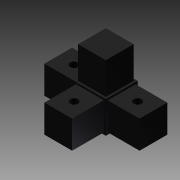
# Autodesk Inventor part: 4-way corner
Saved by Autodesk Inventor 2011 (Build 150239000, 239)
## iProperties
Created: 2013-01-14
Part Number: 4-way corner
Document SubType Name: Modeling
Designer: 351773
Density: 1 g/cm^3
Author: 351773
Autodesk Inventor part; units mm, degrees
ref_plane "YZ Plane" through (0, 0, 0) normal (1, 0, 0) x (0, 1, 0)
ref_plane "XZ Plane" through (0, 0, 0) normal (0, 1, 0) x (-1, 0, 0)
ref_plane "XY Plane" through (0, 0, 0) normal (0, 0, 1) x (1, 0, 0)
sketch "Sketch1" plane through (0, 0, 0) normal (0, 0, 1) x (1, 0, 0)
  line L0 (0, 0) -> (25.4, 0)
  line L1 (25.4, 0) -> (25.4, 25.4)
  line L2 (25.4, 25.4) -> (0, 25.4)
  line L3 (0, 25.4) -> (0, 0)
  line L4 (1.5875, 23.8125) -> (23.8125, 23.8125)
  line L5 (23.8125, 23.8125) -> (23.8125, 1.5875)
  line L6 (23.8125, 1.5875) -> (1.5875, 1.5875)
  line L7 (1.5875, 1.5875) -> (1.5875, 23.8125)
  dimension "d0" = 25.4
  dimension "d1" = 25.4
  dimension "d4" = 1.5875
  constraints: 16 end point, 4 parallel, 2 perpendicular, 1 horizontal, 3 other
  measures "d0" distance of L2.end L1.end
  measures "d1" distance of L1.end L0.end
  measures "d4" distance between parallel lines of L2 L4
extrude "Extrusion1" add sketch "Sketch1" against normal blind 25.4 contours L3 L2 L1 L0 | L4 L5 L6 L7
extrude "Extrusion2" add sketch "Sketch1" along normal blind 25.4 contours L4 L5 L6 L7
sketch "Sketch2" plane through (25.4, 0, 0) normal (1, 0, 0) x (0, 0, -1)
  line L0 (25.4, 0) -> (25.4, 25.4) projected
  line L1 (0, 25.4) -> (25.4, 25.4) projected
  line L2 (0, 0) -> (0, 25.4) projected
  line L3 (0, 0) -> (25.4, 0) projected
  line L4 (23.8125, 23.8125) -> (23.8125, 1.5875)
  line L5 (23.8125, 1.5875) -> (1.5875, 1.5875)
  line L6 (1.5875, 1.5875) -> (1.5875, 23.8125)
  line L7 (1.5875, 23.8125) -> (23.8125, 23.8125)
  dimension "d8" = 1.5875
  constraints: 8 end point, 3 other
  measures "d8" distance between parallel lines of L1 L7
sketch "Sketch3" plane through (0, 25.4, 0) normal (0, 1, 0) x (1, 0, 0)
  line L0 (25.4, 25.4) -> (0, 25.4) projected
  line L1 (0, 0) -> (0, 25.4) projected
  line L2 (25.4, 0) -> (0, 0) projected
  line L3 (25.4, 0) -> (25.4, 25.4) projected
  line L4 (1.5875, 23.8125) -> (23.8125, 23.8125)
  line L5 (23.8125, 23.8125) -> (23.8125, 1.5875)
  line L6 (23.8125, 1.5875) -> (1.5875, 1.5875)
  line L7 (1.5875, 1.5875) -> (1.5875, 23.8125)
  dimension "d9" = 1.5875
  constraints: 8 end point, 3 other
  measures "d9" distance between parallel lines of L0 L4
extrude "Extrusion3" add sketch "Sketch2" along normal blind 25.4 contours L4 L5 L6 L7
extrude "Extrusion4" add sketch "Sketch3" along normal blind 25.4 contours L4 L5 L6 L7
sketch "Sketch4" plane through (0, 0, 0) normal (-1, 0, 0) x (0, 0, 1)
  line L0 (-25.4, 25.4) -> (-25.4, 0) projected
  line L1 (0, 0) -> (-25.4, 0) projected
  line L2 (0, 25.4) -> (0, 0) projected
  line L3 (0, 25.4) -> (-25.4, 25.4) projected
  line L4 (-23.8125, 23.8125) -> (-23.8125, 1.5875)
  line L5 (-23.8125, 1.5875) -> (-1.5875, 1.5875)
  line L6 (-1.5875, 1.5875) -> (-1.5875, 23.8125)
  line L7 (-1.5875, 23.8125) -> (-23.8125, 23.8125)
  dimension "d15" = 1.5875
  constraints: 8 end point, 3 other
  measures "d15" distance between parallel lines of L3 L7
extrude "Extrusion5" add sketch "Sketch4" along normal blind 25.4 contours L7 L6 L5 L4
sketch "Sketch6" plane through (0, 23.8125, -1.5875) normal (0, 1, 0) x (1, 0, 0)
  line L0 (-25.4, 22.225) -> (-25.4, 0) projected
  line L1 (0, 22.225) -> (0, 0) projected
  line L2 (0, 22.225) -> (-25.4, 22.225) projected
  line L3 (25.4, -1.5875) -> (0, -1.5875) projected
  line L4 (0, 0) -> (-25.4, 0) projected
  point P0 (-12.7, 11.1125)
  point P1 (12.7, -14.2875)
  point P2 (38.1, 11.1125)
  dimension "d21" = 12.7
  dimension "d22" = 50.8
  dimension "d23" = 11.1125
  dimension "d24" = 12.7
  dimension "d25" = 12.7
  constraints: 1 horizontal alignment
  measures "d21" distance from line of point (-12.7, 11.113) L0
  measures "d22" distance of point (-12.7, 11.113) point (38.1, 11.113)
  measures "d23" distance from line of L2 point (-12.7, 11.113)
  measures "d24" distance from line of L1 point (12.7, -14.287)
  measures "d25" distance from line of L3 point (12.7, -14.287)
hole "Hole1" at (-12.7, 23.8125, -12.7) at (12.7, 23.8125, 12.7) at (38.1, 23.8125, -12.7) direction (0, -1, 0) diameter 6.35 depth 25.4 tip angle 118
sketch "Sketch7" plane through (23.8125, 25.4, -23.8125) normal (0, 0, -1) x (-1, 0, 0)
  point P0 (23.8125, -25.4)
  point P1 (11.1125, 12.7)
hole "Hole2" at (12.7, 38.1, -23.8125) direction (0, 0, 1) diameter 6.35 depth 25.4 tip angle 118
sketch "Sketch8" plane through (1.5875, 25.4, -23.8125) normal (-1, 0, 0) x (0, 0, 1)
  point P0 (23.8125, -25.4)
  point P1 (11.1125, 12.7)
hole "Hole3" at (1.5875, 38.1, -12.7) direction (1, 0, 0) diameter 6.35 depth 25.4 tip angle 118
body "Solid1"
